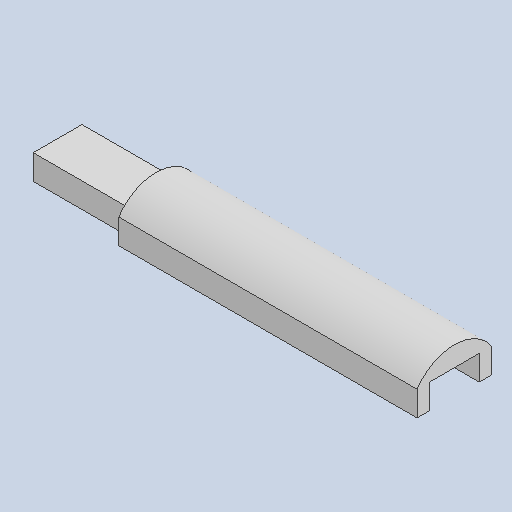
# Autodesk Inventor part: Part_3_hand_extention
Saved by Autodesk Inventor 2023 (Build 270158000, 158)
## iProperties
Created: 2023-09-30
Part Number: Part_3_hand_extention
Material: Generic
Document SubType Name: Modeling
Designer: zskus
Density: 1 g/cm^3
Appearance: Default
Author: zskus
Autodesk Inventor part; units mm, degrees
ref_plane "YZ Plane" through (0, 0, 0) normal (1, 0, 0) x (0, 1, 0)
ref_plane "XZ Plane" through (0, 0, 0) normal (0, 1, 0) x (-1, 0, 0)
ref_plane "XY Plane" through (0, 0, 0) normal (0, 0, 1) x (1, 0, 0)
sketch "Sketch1" plane through (0, 0, 0) normal (0, 1, 0) x (-1, 0, 0)
  line L0 (-38.1, 9.525) -> (38.1, 9.525)
  line L1 (38.1, 9.525) -> (38.1, -9.525)
  line L2 (38.1, -9.525) -> (-38.1, -9.525)
  line L3 (-38.1, -9.525) -> (-38.1, 9.525)
  line L4 (38.1, 6.223) -> (63.246, 6.223)
  line L5 (63.246, 6.223) -> (63.246, -6.223)
  line L6 (63.246, -6.223) -> (38.1, -6.223)
  line L7 (38.1, -6.223) -> (38.1, 6.223)
  point P0 (0, 0)
  point P1 (38.1, 0)
  dimension "d0" = 76.2
  dimension "d1" = 19.05
  dimension "d2" = 9.525
  dimension "d3" = 38.1
  dimension "d4" = 25.146
  dimension "d5" = 12.446
  dimension "d6" = 6.223
  constraints: 16 end point, 4 parallel, 2 horizontal, 2 perpendicular, 1 midpoint, 1 point on line
  measures "d0" distance of L1.end L2.end
  measures "d1" distance of L2.end L0.start
  measures "d2" distance from line of point (0, 0) L2
  measures "d3" distance from line of point (0, 0) L3
  measures "d4" distance of L5.end L6.end
  measures "d5" distance of L4.end L5.end
  measures "d6" distance from line of point (38.1, 0) L6
extrude "Extrusion1" add sketch "Sketch1" along normal blind 6.35
sketch "Sketch2" plane through (38.1, 0, 9.525) normal (1, 0, 0) x (0, 0, -1)
  line L0 (0, 0) -> (19.05, 0) projected
  line L1 (19.05, 0) -> (19.05, 6.35) projected
  line L2 (0, 6.35) -> (19.05, 6.35) projected
  line L3 (0, 0) -> (0, 6.35) projected
  line L4 (19.05, 0) -> (19.05, 6.35) projected
  line L5 (0, 0) -> (0, 6.35) projected
  arc A0 (19.05, 6.35) -> (0, 6.35) centre (9.525, 0) ccw
  point P0 (9.525, 0)
  constraints: 2 point on circle, 1 centre point, 1 coincident
extrude "Extrusion2" add sketch "Sketch2" against normal blind 76.2 contours A0 L2
sketch "Sketch3" plane through (0, 0, 0) normal (0, -1, 0) x (1, 0, 0)
  line L0 (38.1, 9.525) -> (38.1, -9.525) projected
  line L1 (-38.1, 9.525) -> (38.1, 9.525) projected
  line L2 (-38.1, 6.223) -> (-38.1, 9.525) projected
  line L3 (-63.246, 6.223) -> (-38.1, 6.223) projected
  line L4 (-63.246, -6.223) -> (-63.246, 6.223) projected
  line L5 (-38.1, -6.223) -> (-63.246, -6.223) projected
  line L6 (-38.1, -9.525) -> (-38.1, -6.223) projected
  line L7 (38.1, -9.525) -> (-38.1, -9.525) projected
  line L8 (38.1, -9.525) -> (38.1, 9.525) projected
  line L9 (38.1, 6.35) -> (12.7, 6.35)
  line L10 (12.7, 6.35) -> (12.7, -6.35)
  line L11 (12.7, -6.35) -> (38.1, -6.35)
  line L12 (38.1, -6.35) -> (38.1, 6.35)
  point P0 (0, 0)
  point P1 (38.1, 0)
  dimension "d11" = 12.7
  dimension "d12" = 12.446
  dimension "d13" = 6.35
  dimension "d14" = 25.4
  constraints: 8 end point, 2 parallel, 1 horizontal, 1 midpoint, 1 perpendicular, 1 point on line
  measures "d11" distance of L9.end L10.end
  measures "d12" distance between parallel lines of L5 L3
  measures "d13" distance from line of point (38.1, 0) L9
  measures "d14" distance of L9.start L9.end
extrude "Extrusion3" cut sketch "Sketch3" against normal blind 6.35 contours L0 L11 L10 L9
equation "\"d2\" = 0.5 * d1"
equation "\"d3\" = 0.5 * d0"
equation "\"d6\" = 0.5 * d5"
equation "\"d13\" = 0.5 * d11"
body "Solid1"
